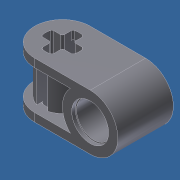
# Autodesk Inventor part: 6536
Saved by Autodesk Inventor 2011 SP2 (Build 150553200, 553)
## iProperties
Company: Allseas Engineering BV
Created: 2011-11-29
Part Number: 6536
Cost Center: 0 kg
Material: Steel
Document SubType Name: Modeling
Designer: PMe
Authority: 0 mm^3
Stock Number: =<Filenr>_<Document number>
Mass: 3.65319 g
Surface Area: 8.52855 cm^2
Volume: 0.465375 cm^3
Density: 7.85 g/cm^3
Act. Code: DW000
SaveDate: 2011-07-28
SaveTime: 18:32
FileName: Standard
TotalMass: 0 kg
TotalVolume: 0 mm^3
Subject: =<Title><TITLE 1_2> <TITLE 2_2>
Author: PMe
Autodesk Inventor part; units mm, degrees
ref_plane "XZ Plane" through (0, 0, 0) normal (0, 1, 0) x (-1, 0, 0)
sketch "Sketch1" plane through (0, 0, 0) normal (0, 0, 1) x (1, 0, 0)
  circle A0 centre (0, 0) radius 4
  dimension "d0" = 8
  constraints: 1 centre point, 1 coincident
  measures "d0" diameter of A0
extrude "Extrusion1" add sketch "Sketch1" along normal mid plane 8
sketch "Sketch2" plane through (0, 0, 4) normal (0, 0, 1) x (1, 0, 0)
  circle A0 centre (0, 0) radius 2.4
  line L0 (-2.2627, 0.8) -> (-0.8, 0.8)
  line L1 (-0.8, 0.8) -> (-0.8, 2.2627)
  line L2 (0.8, 2.2627) -> (0.8, 0.8)
  line L3 (0.8, 0.8) -> (2.2627, 0.8)
  line L4 (2.2627, -0.8) -> (0.8, -0.8)
  line L5 (0.8, -0.8) -> (0.8, -2.2627)
  line L6 (-0.8, -2.2627) -> (-0.8, -0.8)
  line L7 (-0.8, -0.8) -> (-2.2627, -0.8)
  dimension "d3" = 4.8
  dimension "d4" = 1.6
  constraints: 16 end point, 7 equal length, 5 perpendicular, 2 parallel, 1 coincident, 1 horizontal, 10 other
  measures "d4" distance between parallel lines of L5 L6
extrude "Extrusion2" cut sketch "Sketch2" against normal through all contours A0 L4 L5 L6 L7 L0 L1 L2 L3
ref_plane "Work Plane1" through (0, 0, -2.8) normal (0, 0, -1) x (-1, 0, 0)
sketch "Sketch3" plane through (0, 0, -2.8) normal (0, 0, -1) x (-1, 0, 0)
  circle A0 centre (0, 0) radius 4 projected
  circle A1 centre (0, 0) radius 4 projected
  circle A2 centre (0, 0) radius 3
  dimension "d8" = 6
  constraints: 1 centre point, 1 coincident
  measures "d8" diameter of A2
extrude "Extrusion3" cut sketch "Sketch3" against normal blind 5.6
sketch "Sketch5" plane through (0, 0, 0) normal (0, 1, 0) x (-1, 0, 0)
  line L0 (-0.8, 4) -> (-0.8, -4) projected
  line L1 (0.8, 4) -> (0.8, -4) projected
  line L2 (4, 2.8) -> (-4, 2.8) projected
  line L3 (-0.8, -2.8) -> (0.8, -2.8)
  line L4 (0.8, -2.8) -> (0.8, 2.8)
  line L5 (0.8, 2.8) -> (-0.8, 2.8)
  line L6 (-0.8, 2.8) -> (-0.8, -2.8)
  point P0 (0, 0)
  point P1 (-1.518, -3.6)
  point P2 (4, -2.8)
  point P3 (4, -2.8)
  constraints: 8 end point, 3 point on line, 2 parallel, 1 horizontal, 1 perpendicular, 2 other
extrude "Extrusion5" cut sketch "Sketch5" along normal through all both and the other way through all
fillet "Fillet1" radius 0.3 16 edges at (-0.8, 0.8, 0) (-0.8, -0.8, 0) (0.8, -0.8, 0) (0.8, 0.8, 0) (-2.2627, -0.8, 0) (-2.2627, 0.8, 0) (-0.8, 2.2627, 3.4) (0.8, 2.2627, 3.4) (2.2627, 0.8, 0) (2.2627, -0.8, 0) (0.8, -2.2627, 3.4) (-0.8, -2.2627, 3.4) (0.8, 2.2627, -3.4) (-0.8, 2.2627, -3.4) (0.8, -2.2627, -3.4) (-0.8, -2.2627, -3.4)
sketch "Sketch6" plane through (0, 0, 0) normal (0, 1, 0) x (-1, 0, 0)
  circle A0 centre (-8, 0) radius 2.5
  circle A1 centre (-8, 0) radius 4
  line L0 (-4, 2.8) -> (-4, 4)
  line L1 (-4, -4) -> (-4, -2.8)
  line L2 (-8, 4) -> (-8, -4) construction
  point P0 (0, 0)
  dimension "d22" = 5
  dimension "d23" = 8
  dimension "d24" = 8
  constraints: 6 end point, 2 centre point, 2 point on circle, 1 coincident, 1 horizontal alignment, 1 midpoint, 1 parallel
  measures "d22" diameter of A0
  measures "d23" diameter of A1
  measures "d24" distance of point (0, 0) A0.centre
extrude "Extrusion6" add sketch "Sketch6" along normal mid plane 8
sketch "Sketch7" plane through (8, 4, 0) normal (0, 1, 0) x (1, 0, 0)
  circle A0 centre (0, 0) radius 2.5 projected
  circle A1 centre (0, 0) radius 4 projected
  circle A2 centre (0, 0) radius 2.6667
  point P0 (-8, 0)
  dimension "d27" = 5.3333
  constraints: 1 centre point, 1 coincident
  measures "d27" diameter of A2
extrude "Extrusion7" cut sketch "Sketch7" against normal blind 0.5333 contours A2
mirror "Mirror1" about plane through (0, 0, 0) normal (0, 1, 0) of "Extrusion7"
ref_plane "Work Plane2" through (8, 0, 0) normal (1, 0, 0) x (0, 1, 0)
sketch "Sketch8" plane through (8, 0, 0) normal (1, 0, 0) x (0, 1, 0)
  line L0 (-4, -2.6667) -> (-4, 2.6667) projected
  line L1 (-4, -4) -> (-4, 4) projected
  line L2 (4, 2.6667) -> (4, -2.6667) projected
  line L3 (4, 4) -> (4, -4) projected
  line L4 (4, 4) -> (-4, 4)
  line L5 (-4, 4) -> (-4, 2.8)
  line L6 (-4, 2.8) -> (4, 2.8)
  line L7 (4, 2.8) -> (4, 4)
  line L8 (-4, -4) -> (4, -4)
  line L9 (4, -4) -> (4, -2.8)
  line L10 (4, -2.8) -> (-4, -2.8)
  line L11 (-4, -2.8) -> (-4, -4)
  dimension "d36" = 1.2
  constraints: 16 end point, 4 parallel, 2 horizontal, 2 perpendicular, 2 point on line, 1 collinear
  measures "d36" distance between parallel lines of L8 L10
extrude "Extrusion8" add sketch "Sketch8" against normal up to surface contours L10 L3 L8 L1 | L1 L4 L3 L6
body "Solid1"
